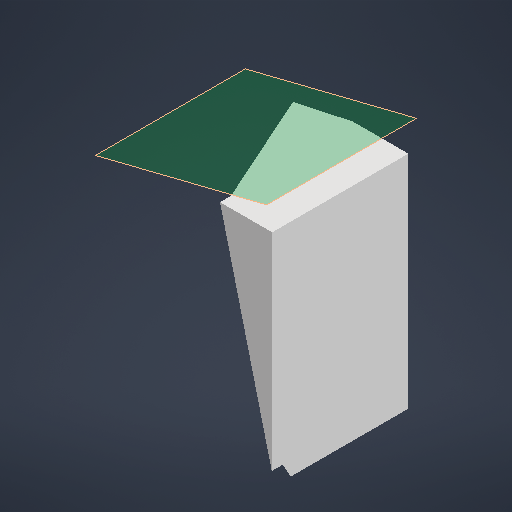
# Autodesk Inventor part: Lid
Saved by Autodesk Inventor 2026 (Build 300175050, 175E)
## iProperties
Created: 2026-06-21
Part Number: Lid
Material: Generic
Document SubType Name: Modeling
Designer: sniel
Density: 1 g/cm^3
Appearance: Default
Author: sniel
Autodesk Inventor part; units mm, degrees
ref_plane "YZ Plane" through (0, 0, 0) normal (1, 0, 0) x (0, 1, 0)
ref_plane "XZ Plane" through (0, 0, 0) normal (0, 1, 0) x (-1, 0, 0)
ref_plane "XY Plane" through (0, 0, 0) normal (0, 0, 1) x (1, 0, 0)
sketch "Sketch1" plane through (0, 0, 0) normal (0, 0, 1) x (1, 0, 0)
  line L0 (43.3243, -30.319) -> (27.0819, 34.6507)
  line L1 (43.6847, -30.319) -> (43.3243, -30.319)
  line L2 (43.8153, 34.6507) -> (43.6847, -30.319)
  line L3 (27.0819, 34.6507) -> (43.8153, 34.6507)
  point P0 (0, 0)
  constraints: 8 end point
extrude "Extrusion1" add sketch "Sketch1" along normal blind 40
sketch "Sketch2" plane through (0, 0, 40) normal (0, 0, 1) x (1, 0, 0)
  line L0 (43.6847, -30.319) -> (43.8153, 34.6507)
  line L1 (43.8153, 34.6507) -> (27.0819, 34.6507)
  line L2 (27.0819, 34.6507) -> (43.3243, -30.319)
  line L3 (43.3243, -30.319) -> (43.6847, -30.319)
  line L4 (9.5067, 30.2569) -> (11.5067, 30.2569)
  line L5 (11.5067, 30.2569) -> (11.5067, 34.6507)
  line L6 (11.5067, 34.6507) -> (27.0819, 34.6507)
  line L7 (11.5067, 34.6507) -> (43.3243, -30.319)
  point P0 (0, 0)
  dimension "d2" = 2
  constraints: 16 end point
  measures "d2" distance of L4.start L4.end
extrude "Extrusion2" add sketch "Sketch2" against normal blind 40 contours L7 L6 L2
sketch "Sketch3" plane through (0, 0, 0) normal (0, 0, -1) x (-1, 0, 0)
  line L0 (-43.6847, -30.319) -> (-43.8153, 34.6507) projected
  line L1 (-43.3243, -30.319) -> (-43.6847, -30.319) projected
  line L2 (-43.3243, -30.319) -> (-11.5067, 34.6507) projected
  line L3 (-43.8153, 34.6507) -> (-11.5067, 34.6507) projected
  arc A0 (-11.5067, 34.6507) -> (-43.3243, -30.319) centre (56.3122, -38.8381) ccw
  point P0 (0, 0)
  dimension "d5" = 100
  constraints: 2 point on circle, 1 centre point
  measures "d5" radius of A0
extrude "Extrusion3" cut sketch "Sketch3" against normal blind 40 contours A0 L2
ref_plane "Work Plane1" through (25.8481, -31.3143, 21.5224) normal (0.9701425, 0.2425356, 0) x (0, 0, -1)
ref_plane "Work Plane4" through (11.5067, 34.6507, 40) normal (0.2425356, -0.9701425, 0) x (0, 0, -1)
ref_plane "Work Plane3" through (25.8481, -31.3143, 21.5224) normal (0.9701425, 0.2425356, 0) x (0, 0, -1)
sketch "Sketch5" plane through (11.5067, 34.6507, 40) normal (0.2425356, -0.9701425, 0) x (0, 0, -1)
  line L0 (29.9641, 1.0219) -> (3.228, 13.4892)
  line L1 (3.228, 13.4892) -> (3.228, 16.4892)
  line L2 (3.228, 16.4892) -> (0, 16.4892)
  line L3 (0, 31.344) -> (0, 0) projected
  line L4 (40, 31.344) -> (40, 0) projected
  line L5 (0, 0) -> (40, 0) projected
  line L6 (0, 31.344) -> (0, 0) projected
  line L7 (40, 31.344) -> (0, 31.344) projected
  line L8 (29.9641, 1.0219) -> (40, 1.0219)
  arc A0 (36.6954, 1.9144) -> (36.6283, 1.4007) centre (38.6283, 1.4007) ccw projected
  line L9 (36.6954, 1.9144) -> (40, 1.9144) projected
  line L10 (40, 1.9144) -> (40, -5.9625) projected
  arc A1 (40, -5.9625) -> (38.4823, -3.5717) centre (32.6454, -8.9542) ccw projected
  arc A2 (36.6283, 1.1737) -> (38.4823, -3.5717) centre (43.6283, 1.1737) ccw projected
  line L11 (36.6283, 1.1737) -> (36.6283, 1.4007) projected
  arc A3 (36.867, 2.3482) -> (36.6954, 1.9144) centre (38.6283, 1.4007) ccw projected
  arc A4 (36.867, 2.3482) -> (40, 14.7848) centre (13.75, 14.7848) ccw projected
  line L12 (40, 14.7848) -> (40, 31.0187) projected
  line L13 (44.6283, 31.0187) -> (40, 31.0187) projected
  line L14 (44.6283, -24.8913) -> (44.6283, 31.0187) projected
  line L15 (44.6283, -24.8913) -> (40, -24.8913) projected
  line L16 (40, -24.8913) -> (40, 1.9144) projected
  line L17 (36.6954, 1.9144) -> (40, 1.9144) projected
  line L18 (36.6954, 1.9144) -> (3.228, 16.4892)
  line L19 (40, 15.4598) -> (40, 31.344) projected
  line L20 (40, 14.7848) -> (40, 15.4598)
  line L21 (40, 15.4598) -> (0, 15.4598) projected
  line L22 (40, 15.4598) -> (36.1857, 2.1363)
  point P0 (40, -19.5671)
  point P1 (0, 0)
  point P2 (36.7274, 0)
  dimension "d10" = 3
  constraints: 14 end point, 3 point on line, 1 collinear, 1 horizontal, 1 perpendicular, 1 vertical
  measures "d10" distance of L0.end L1.end
extrude "Extrusion4" cut sketch "Sketch5" along normal blind 72.5 contours L8 A2 L5 L3 L21 L1 L0 | L0 L1 L21 L18 A0 L11 A2 L8 | A2 L11 A0 L9 L4 L8 | L8 L4 L5 A2 | L21 L3 L2 L1 | L1 L18 L21 | L5 L10 A1 A2 | L9 A3 A4 L4 | L22 L4 A4 A3 L18
body "Solid1"
